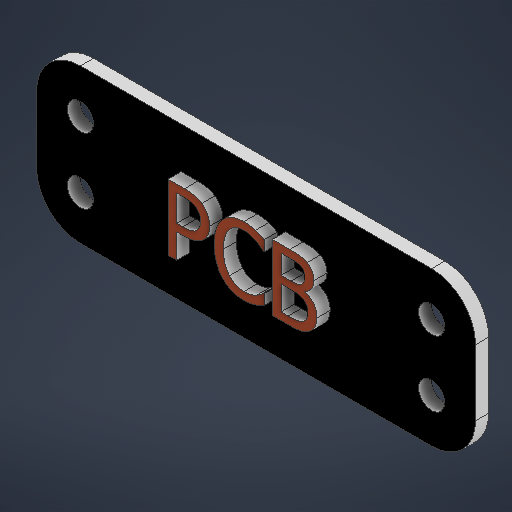
# Autodesk Inventor part: PCB
Saved by Autodesk Inventor 2025 (Build 290162000, 162)
## iProperties
Created: 2024-05-23
Part Number: PCB
Material: Generic
Document SubType Name: Modeling
Designer: techn
Density: 1 g/cm^3
Appearance: Default
Author: techn
Autodesk Inventor part; units mm, degrees
ref_plane "YZ Plane" through (0, 0, 0) normal (1, 0, 0) x (0, 1, 0)
ref_plane "XZ Plane" through (0, 0, 0) normal (0, 1, 0) x (-1, 0, 0)
ref_plane "XY Plane" through (0, 0, 0) normal (0, 0, 1) x (1, 0, 0)
sketch "Sketch1" plane through (0, 0, 0) normal (0, 0, 1) x (1, 0, 0)
  circle A0 centre (0, 0) radius 1.5
  circle A1 centre (0, 0) radius 3
  circle A2 centre (0, 15) radius 1.5
  circle A3 centre (0, 15) radius 3
  circle A4 centre (80, 15) radius 1.5
  circle A5 centre (80, 15) radius 3
  circle A6 centre (80, 0) radius 1.5
  circle A7 centre (80, 0) radius 3
  line L0 (0, 25) -> (80, 25)
  line L1 (90, 15) -> (90, 0)
  line L2 (80, -10) -> (0, -10)
  line L3 (-10, 0) -> (-10, 15)
  arc A8 (0, 25) -> (-10, 15) centre (0, 15) ccw
  arc A9 (-10, 0) -> (0, -10) centre (0, 0) ccw
  arc A10 (80, -10) -> (90, 0) centre (80, 0) ccw
  arc A11 (90, 15) -> (80, 25) centre (80, 15) ccw
  dimension "d0" = 3
  dimension "d1" = 1.5
  dimension "d2" = 3
  dimension "d3" = 1.5
  dimension "d4" = 3
  dimension "d5" = 1.5
  dimension "d6" = 3
  dimension "d7" = 1.5
  dimension "d8" = 80
  dimension "d9" = 15
  dimension "d10" = 10
  dimension "d11" = 10
  dimension "d12" = 10
  dimension "d13" = 10
  dimension "d14" = 10
  constraints: 12 centre point, 8 end point, 8 point on circle, 8 tangent, 3 equal radius, 2 horizontal alignment, 2 parallel, 2 vertical alignment, 1 coincident, 1 horizontal, 1 perpendicular
  measures "d0" diameter of A0
  measures "d1" radial gap between concentric circles of A0 A1
  measures "d2" diameter of A2
  measures "d3" radial gap between concentric circles of A2 A3
  measures "d4" diameter of A4
  measures "d5" radial gap between concentric circles of A4 A5
  measures "d6" diameter of A6
  measures "d7" radial gap between concentric circles of A6 A7
  measures "d8" distance of A6.centre A0.centre
  measures "d9" distance of A0.centre A2.centre
  measures "d10" distance from line of L3 A2.centre
  measures "d11" distance from line of L0 A2.centre
  measures "d12" distance from line of L2 A0.centre
  measures "d13" distance from line of L1 A6.centre
  measures "d14" radius of A8
extrude "Extrusion1" add sketch "Sketch1" along normal blind 3 contours L0 A11 L1 A10 L2 A9 L3 A8
sketch "Sketch2" plane through (0, 0, 3) normal (0, 0, 1) x (1, 0, 0)
  line L0 (21.4385, 15.8987) -> (36.0458, 15.8987) construction
  line L1 (36.0458, 15.8987) -> (36.0458, 9.5812) construction
  line L2 (36.0458, 9.5812) -> (21.4385, 9.5812) construction
  line L3 (21.4385, 9.5812) -> (21.4385, 15.8987) construction
  spline S0 degree 2 poles (32.4393, 11.1094) (32.4393, 10.137) (31.7464, 8.3866) (31.1265, 7.7788) knots 0 0 0 1 2 2 2
  spline S1 degree 2 poles (31.1265, 7.7788) (30.3485, 7.013) (28.2456, 6.2229) (26.6411, 6.2229) knots 0 0 0 1 2 2 2
  line L4 (26.6411, 6.2229) -> (24.9514, 6.2229)
  line L5 (24.9514, 6.2229) -> (24.9514, 0.6313)
  line L6 (24.9514, 0.6313) -> (22.9579, 0.6313)
  line L7 (22.9579, 0.6313) -> (22.9579, 15.6313)
  line L8 (22.9579, 15.6313) -> (26.7261, 15.6313)
  spline S2 degree 2 poles (26.7261, 15.6313) (28.0633, 15.6313) (29.9352, 15.1937) (30.6524, 14.6953) knots 0 0 0 1 2 2 2
  spline S3 degree 2 poles (30.6524, 14.6953) (31.4911, 14.124) (32.4393, 12.3615) (32.4393, 11.1094) knots 0 0 0 1 2 2 2
  spline S4 degree 2 poles (30.3607, 11.0487) (30.3607, 11.8266) (29.8258, 12.9692) (29.2788, 13.3339) knots 0 0 0 1 2 2 2
  spline S5 degree 2 poles (29.2788, 13.3339) (28.8048, 13.65) (27.5406, 13.9052) (26.6046, 13.9052) knots 0 0 0 1 2 2 2
  line L9 (26.6046, 13.9052) -> (24.9514, 13.9052)
  line L10 (24.9514, 13.9052) -> (24.9514, 7.9247)
  line L11 (24.9514, 7.9247) -> (26.3129, 7.9247)
  spline S6 degree 2 poles (26.3129, 7.9247) (27.5284, 7.9247) (29.0236, 8.3137) (29.5098, 8.8242) knots 0 0 0 1 2 2 2
  spline S7 degree 2 poles (29.5098, 8.8242) (29.9595, 9.2739) (30.3607, 10.3315) (30.3607, 11.0487) knots 0 0 0 1 2 2 2
  spline S8 degree 2 poles (40.1945, 0.3639) (38.7359, 0.3639) (36.2683, 1.3485) (35.3688, 2.3331) knots 0 0 0 1 2 2 2
  spline S9 degree 2 poles (35.3688, 2.3331) (34.4693, 3.3056) (33.4847, 6.2229) (33.4847, 8.1192) knots 0 0 0 1 2 2 2
  spline S10 degree 2 poles (33.4847, 8.1192) (33.4847, 10.0033) (34.4449, 12.7991) (35.3566, 13.8323) knots 0 0 0 1 2 2 2
  spline S11 degree 2 poles (35.3566, 13.8323) (36.2561, 14.8412) (38.7116, 15.8987) (40.231, 15.8987) knots 0 0 0 1 2 2 2
  spline S12 degree 2 poles (40.231, 15.8987) (40.9847, 15.8987) (42.3096, 15.6799) (42.8688, 15.5098) knots 0 0 0 1 2 2 2
  spline S13 degree 2 poles (42.8688, 15.5098) (43.355, 15.3517) (44.3639, 14.902) (44.8623, 14.6346) knots 0 0 0 1 2 2 2
  line L12 (44.8623, 14.6346) -> (44.8623, 12.2278)
  line L13 (44.8623, 12.2278) -> (44.7043, 12.2278)
  spline S14 degree 2 poles (44.7043, 12.2278) (44.4368, 12.4709) (43.6103, 13.1516) (43.0146, 13.4798) knots 0 0 0 1 2 2 2
  spline S15 degree 2 poles (43.0146, 13.4798) (42.4433, 13.7958) (41.0941, 14.197) (40.2189, 14.197) knots 0 0 0 1 2 2 2
  spline S16 degree 2 poles (40.2189, 14.197) (39.2586, 14.197) (37.5446, 13.4068) (36.9004, 12.6532) knots 0 0 0 1 2 2 2
  spline S17 degree 2 poles (36.9004, 12.6532) (36.2683, 11.8874) (35.5633, 9.5657) (35.5633, 8.1192) knots 0 0 0 1 2 2 2
  spline S18 degree 2 poles (35.5633, 8.1192) (35.5633, 6.5754) (36.3048, 4.3509) (36.949, 3.5851) knots 0 0 0 1 2 2 2
  spline S19 degree 2 poles (36.949, 3.5851) (37.5811, 2.8436) (39.2707, 2.09) (40.2189, 2.09) knots 0 0 0 1 2 2 2
  spline S20 degree 2 poles (40.2189, 2.09) (41.0819, 2.09) (42.5527, 2.5154) (43.124, 2.8315) knots 0 0 0 1 2 2 2
  spline S21 degree 2 poles (43.124, 2.8315) (43.671, 3.1475) (44.4855, 3.8039) (44.7164, 4.0349) knots 0 0 0 1 2 2 2
  line L14 (44.7164, 4.0349) -> (44.8623, 4.0349)
  line L15 (44.8623, 4.0349) -> (44.8623, 1.6524)
  spline S22 degree 2 poles (44.8623, 1.6524) (44.3639, 1.4214) (43.4887, 0.996) (42.8688, 0.8015) knots 0 0 0 1 2 2 2
  spline S23 degree 2 poles (42.8688, 0.8015) (42.2124, 0.5827) (41.0941, 0.3639) (40.1945, 0.3639) knots 0 0 0 1 2 2 2
  spline S24 degree 2 poles (56.8963, 5.2383) (56.8963, 4.12) (56.0454, 2.406) (55.3404, 1.8469) knots 0 0 0 1 2 2 2
  spline S25 degree 2 poles (55.3404, 1.8469) (54.4895, 1.1905) (52.5568, 0.6313) (51.0252, 0.6313) knots 0 0 0 1 2 2 2
  line L16 (51.0252, 0.6313) -> (46.7221, 0.6313)
  line L17 (46.7221, 0.6313) -> (46.7221, 15.6313)
  line L18 (46.7221, 15.6313) -> (50.697, 15.6313)
  spline S26 degree 2 poles (50.697, 15.6313) (52.3015, 15.6313) (53.9061, 15.4247) (54.6354, 15.0235) knots 0 0 0 1 2 2 2
  spline S27 degree 2 poles (54.6354, 15.0235) (55.4498, 14.5981) (56.1913, 13.2002) (56.1913, 12.2521) knots 0 0 0 1 2 2 2
  spline S28 degree 2 poles (56.1913, 12.2521) (56.1913, 11.1945) (55.073, 9.5171) (54.0884, 9.043) knots 0 0 0 1 2 2 2
  line L19 (54.0884, 9.043) -> (54.0884, 8.9701)
  spline S29 degree 2 poles (54.0884, 8.9701) (55.4255, 8.6054) (56.8963, 6.6727) (56.8963, 5.2383) knots 0 0 0 1 2 2 2
  spline S30 degree 2 poles (54.8177, 5.1532) (54.8177, 6.0041) (54.3315, 7.0981) (53.6022, 7.4871) knots 0 0 0 1 2 2 2
  spline S31 degree 2 poles (53.6022, 7.4871) (53.1281, 7.7302) (52.0098, 7.8761) (50.9766, 7.8761) knots 0 0 0 1 2 2 2
  line L20 (50.9766, 7.8761) -> (48.7156, 7.8761)
  line L21 (48.7156, 7.8761) -> (48.7156, 2.3331)
  line L22 (48.7156, 2.3331) -> (50.3323, 2.3331)
  spline S32 degree 2 poles (50.3323, 2.3331) (51.6451, 2.3331) (53.1524, 2.5762) (53.7359, 2.9652) knots 0 0 0 1 2 2 2
  spline S33 degree 2 poles (53.7359, 2.9652) (54.295, 3.3663) (54.8177, 4.3631) (54.8177, 5.1532) knots 0 0 0 1 2 2 2
  spline S34 degree 2 poles (54.1127, 11.9725) (54.1127, 12.5073) (53.748, 13.3096) (53.3469, 13.5406) knots 0 0 0 1 2 2 2
  spline S35 degree 2 poles (53.3469, 13.5406) (52.8607, 13.808) (51.6816, 13.9295) (50.624, 13.9295) knots 0 0 0 1 2 2 2
  line L23 (50.624, 13.9295) -> (48.7156, 13.9295)
  line L24 (48.7156, 13.9295) -> (48.7156, 9.5414)
  line L25 (48.7156, 9.5414) -> (50.9766, 9.5414)
  spline S36 degree 2 poles (50.9766, 9.5414) (51.9125, 9.5414) (52.7999, 9.7359) (53.274, 10.0398) knots 0 0 0 1 2 2 2
  spline S37 degree 2 poles (53.274, 10.0398) (53.7359, 10.3315) (54.1127, 11.2675) (54.1127, 11.9725) knots 0 0 0 1 2 2 2
  point P0 (0, 0)
  dimension "d7" = 1.5
  constraints: 2 other
extrude "Extrusion2" add sketch "Sketch2" along normal blind 3
body "Solid1"
